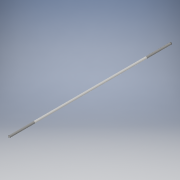
# Autodesk Inventor part: Axle
Saved by Autodesk Inventor 2019 (Build 230136000, 136)
## iProperties
Created: 2020-01-15
Part Number: Axle
Material: Generic
Document SubType Name: Modeling
Designer: 18186
Density: 1 g/cm^3
Appearance: Default
Author: 18186
Autodesk Inventor part; units mm, degrees
ref_plane "YZ Plane" through (0, 0, 0) normal (1, 0, 0) x (0, 1, 0)
ref_plane "XZ Plane" through (0, 0, 0) normal (0, 1, 0) x (-1, 0, 0)
sketch "Sketch3" plane through (0, 0, 0) normal (0, 0, 1) x (1, 0, 0)
  circle A0 centre (0, 0) radius 4.5
  dimension "d5" = 9
  constraints: 1 centre point, 1 coincident
  measures "d5" diameter of A0
extrude "Extrusion3" add sketch "Sketch3" along normal blind 114.3
ref_plane "Work Plane2" through (0, 0, -127) normal (0, 0, -1) x (-1, 0, 0)
mirror "Mirror1" about plane through (0, 0, -127) normal (0, 0, -1) of "Extrusion3"
sketch "Sketch5" plane through (0, 0, -127) normal (0, 0, -1) x (-1, 0, 0)
  circle A0 centre (0, 0) radius 4.5
  constraints: 1 centre point, 1 coincident
extrude "Extrusion4" add sketch "Sketch5" along normal mid plane 254
sketch "Sketch6" plane through (0, 0, 114.3) normal (0, 0, 1) x (1, 0, 0)
  circle A0 centre (0, 0) radius 4.5
  constraints: 1 centre point, 1 coincident
extrude "Extrusion5" add sketch "Sketch6" along normal blind 121.92
sketch "Sketch7" plane through (0, 0, -368.3) normal (0, 0, -1) x (-1, 0, 0)
  circle A0 centre (0, 0) radius 4.5
  constraints: 1 centre point, 1 coincident
extrude "Extrusion6" add sketch "Sketch7" along normal blind 121.92
thread "Thread3" size "3/8-16 UNC" class "2A" standard "ANSI Unified Screw Threads" length 111.76
thread "Thread4" size "3/8-16 UNC" class "2A" standard "ANSI Unified Screw Threads" length 111.76
body "Solid2"
